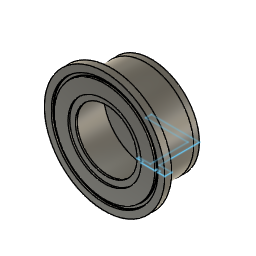
Desgin A Base (Autodesk Fusion 360 design; units mm, degrees)
Autodesk Fusion 360 part; units mm, degrees
note: some values were not read from the file. Set by a fixed rule: which sketch regions a step uses.
sketch "Sketch1" plane through (0, 0, 0) normal (0, 0, 1) x (1, 0, 0)
  line L0 (52.6987, 6) -> (52.6987, 0)
  line L1 (46.7394, -0.0003) -> (46.7394, 1.3197)
  line L2 (43.9694, 1.3205) -> (43.9694, 0.0001)
  line L3 (46.7394, -0.0003) -> (52.6987, 0)
  line L4 (36.9987, 6.0005) -> (37.0139, 3.0519)
  line L5 (37.0139, 3.0519) -> (26.9987, 3.0003)
  line L6 (36.9987, 6.0005) -> (36.9385, 36.0005)
  line L7 (41.9385, 36.0005) -> (41.9987, 6.0003)
  line L8 (41.9385, 36.0005) -> (41.9521, 41.0005)
  line L9 (41.9521, 41.0005) -> (34.7652, 41.0204)
  line L10 (41.9987, 6.0003) -> (52.6987, 6)
  line L11 (26.9987, 1.5) -> (31.9987, 1.5)
  line L12 (31.9987, 1.5) -> (31.9994, 0)
  line L13 (26.9987, 1.5) -> (26.9987, 3.0003)
  line L14 (43.9694, 1.3205) -> (43.9694, 1.8205)
  line L15 (46.7394, 1.3197) -> (46.7394, 1.8197)
  line L16 (43.9694, 1.8205) -> (46.7394, 1.8197)
  line L17 (36.9385, 36.0005) -> (0, 36.0005)
  line L18 (34.7652, 41.0204) -> (0, 41.0204)
  line L19 (0, 36.0005) -> (0, 41.0204)
  line L20 (43.9694, 0.0001) -> (31.9994, 0)
  dimension "d35" = 5
  dimension "d38" = 5
  dimension "d40" = 5
  dimension "d43" = 0.5
  dimension "d44" = 0.5
  constraint parallel L2 L14
  constraint parallel L1 L15
  constraint perpendicular L18 L19
  measures "d35" distance of L6.end L7.start
  measures "d38" distance of L7.start L8.end
  measures "d40" distance of L11.start L11.end
  measures "d43" distance of L2.start L14.end
  measures "d44" distance of L1.end L15.end
revolve "Revolve1" add sketch "Sketch1" angle 360 about axis through (0, 1.75, 0) along (0, 1, 0) makes body 1
fillet "Fillet5" radius 0.3 1 edges at (-43.5764, 1.8197, -16.9017) on bodies 1
fillet "Fillet6" radius 0.3 1 edges at (-40.9938, 1.8205, -15.9) on bodies 1
sketch "Sketch2" plane through (0, 0, 0) normal (0, 1, 0) x (1, 0, 0)
  circle A0 centre (0, 0) radius 31
  circle A1 centre (0, -5) radius 1.5
  circle A2 centre (0, -10) radius 1.5
  circle A3 centre (0, -15) radius 1.5
  circle A4 centre (0, -20) radius 1.5
  circle A5 centre (4.3301, -2.5) radius 1.5
  circle A6 centre (4.3301, 2.5) radius 1.5
  circle A7 centre (0, 5) radius 1.5
  circle A8 centre (-4.3301, 2.5) radius 1.5
  circle A9 centre (-4.3301, -2.5) radius 1.5
  circle A10 centre (5.8779, -8.0902) radius 1.5
  circle A11 centre (9.5106, -3.0902) radius 1.5
  circle A12 centre (9.5106, 3.0902) radius 1.5
  circle A13 centre (5.8779, 8.0902) radius 1.5
  circle A14 centre (0, 10) radius 1.5
  circle A15 centre (-5.8779, 8.0902) radius 1.5
  circle A16 centre (-9.5106, 3.0902) radius 1.5
  circle A17 centre (-9.5106, -3.0902) radius 1.5
  circle A18 centre (-5.8779, -8.0902) radius 1.5
  circle A19 centre (6.5083, -13.5145) radius 1.5
  circle A20 centre (11.7275, -9.3523) radius 1.5
  circle A21 centre (14.6239, -3.3378) radius 1.5
  circle A22 centre (14.6239, 3.3378) radius 1.5
  circle A23 centre (11.7275, 9.3523) radius 1.5
  circle A24 centre (6.5083, 13.5145) radius 1.5
  circle A25 centre (0, 15) radius 1.5
  circle A26 centre (-6.5083, 13.5145) radius 1.5
  circle A27 centre (-11.7275, 9.3523) radius 1.5
  circle A28 centre (-14.6239, 3.3378) radius 1.5
  circle A29 centre (-14.6239, -3.3378) radius 1.5
  circle A30 centre (-11.7275, -9.3523) radius 1.5
  circle A31 centre (-6.5083, -13.5145) radius 1.5
  circle A32 centre (6.8404, -18.7939) radius 1.5
  circle A33 centre (12.8558, -15.3209) radius 1.5
  circle A34 centre (17.3205, -10) radius 1.5
  circle A35 centre (19.6962, -3.473) radius 1.5
  circle A36 centre (19.6962, 3.473) radius 1.5
  circle A37 centre (17.3205, 10) radius 1.5
  circle A38 centre (12.8558, 15.3209) radius 1.5
  circle A39 centre (6.8404, 18.7939) radius 1.5
  circle A40 centre (0, 20) radius 1.5
  circle A41 centre (-6.8404, 18.7939) radius 1.5
  circle A42 centre (-12.8558, 15.3209) radius 1.5
  circle A43 centre (-17.3205, 10) radius 1.5
  circle A44 centre (-19.6962, 3.473) radius 1.5
  circle A45 centre (-19.6962, -3.473) radius 1.5
  circle A46 centre (-17.3205, -10) radius 1.5
  circle A47 centre (-12.8558, -15.3209) radius 1.5
  circle A48 centre (-6.8404, -18.7939) radius 1.5
  circle A49 centre (0, 0) radius 1.5
  dimension "d49" = 62
  dimension "d50" = 5
  dimension "d51" = 3
  dimension "d52" = 5
  dimension "d53" = 3
  dimension "d54" = 5
  dimension "d55" = 3
  dimension "d56" = 5
  dimension "d57" = 3
  dimension "d59" = 360
  dimension "d61" = 360
  dimension "d63" = 360
  dimension "d65" = 360
  dimension "d66" = 3
  constraint coincident A0.centre A49.centre
  constraint concentric A0 A49
  measures "d49" diameter of A0
  measures "d50" distance of A0.centre A1.centre
  measures "d51" diameter of A1
  measures "d52" distance of A1.centre A2.centre
  measures "d53" diameter of A2
  measures "d54" distance of A2.centre A3.centre
  measures "d55" diameter of A3
  measures "d56" distance of A3.centre A4.centre
  measures "d57" diameter of A4
  measures "d66" diameter of A49
extrude "Extrude1" add sketch "Sketch2" against normal blind 1 separate body makes body 2
hidden bodies 2
